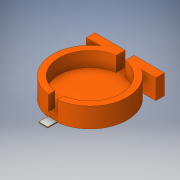
# Autodesk Inventor part: Keystone1056_12_5mmCoinCell
Saved by Autodesk Inventor 2016 (Build 200138000, 138)
## iProperties
Created: 2016-09-29
Part Number: Keystone1056_12_5mmCoinCell
Material: Generic
Document SubType Name: Modeling
Designer: jfixelle
Density: 1 g/cm^3
Appearance: Smooth - Light Orange
Author: jfixelle
Autodesk Inventor part; units mm, degrees
ref_plane "YZ Plane" through (0, 0, 0) normal (1, 0, 0) x (0, 1, 0)
ref_plane "XZ Plane" through (0, 0, 0) normal (0, 1, 0) x (-1, 0, 0)
ref_plane "XY Plane" through (0, 0, 0) normal (0, 0, 1) x (1, 0, 0)
sketch "Sketch1" plane through (0, 0, 0) normal (0, 1, 0) x (-1, 0, 0)
  arc A0 (4.1548, -6.25) -> (-4.1548, -6.25) centre (0, 0) ccw
  circle A1 centre (0, 0) radius 6.25 construction
  line L0 (-7, -6.25) -> (-7, -7.985)
  line L1 (-7, -7.985) -> (7, -7.985)
  line L2 (7, -7.985) -> (7, -6.25)
  line L3 (0, 7.505) -> (-2.894, 7.505)
  line L4 (7, -6.25) -> (4.1548, -6.25)
  line L5 (-4.1548, -6.25) -> (-7, -6.25)
  dimension "d0" = 15.01
  dimension "d1" = 12.5
  dimension "d2" = 15.49
  dimension "d4" = 14
  dimension "d5" = 7
  constraints: 12 end point, 3 horizontal, 3 parallel, 3 point on circle, 2 centre point, 2 coincident, 2 perpendicular, 1 tangent
  measures "d0" diameter of A0
  measures "d1" diameter of A1
  measures "d2" distance between parallel lines of L1 L3
  measures "d4" distance of L0.end L1.end
  measures "d5" distance from line of point (0, 0) L2
extrude "Extrusion1" add sketch "Sketch1" along normal blind 4
sketch "Sketch2" plane through (0, 4, 0) normal (0, 1, 0) x (1, 0, 0)
  circle A0 centre (0, 0) radius 6.25
  line L0 (-0.9, -7.9572) -> (0.9, -7.9572)
  line L1 (0.9, -7.9572) -> (0.9, 8.949)
  line L2 (0.9, 8.949) -> (-0.9, 8.949)
  line L3 (-0.9, 8.949) -> (-0.9, -7.9572)
  dimension "d8" = 12.5
  dimension "d11" = 1.8
  dimension "d12" = 0.9
  constraints: 8 end point, 2 parallel, 1 centre point, 1 coincident, 1 horizontal, 1 perpendicular
  measures "d8" diameter of A0
  measures "d11" distance of L0.start L0.end
  measures "d12" distance from line of point (0, 0) L3
extrude "Extrusion2" cut sketch "Sketch2" against normal blind 3
sketch "Sketch3" plane through (0, 0, 0) normal (0, -1, 0) x (1, 0, 0)
  line L0 (0.9, 5.5692) -> (-0.9, 5.5692)
  line L1 (-0.9, 5.5692) -> (-0.9, 9.4)
  line L2 (-0.9, 9.4) -> (0.9, 9.4)
  line L3 (0.9, 9.4) -> (0.9, 5.5692)
  line L4 (-0.9, -6.2525) -> (0.9, -6.2525)
  line L5 (0.9, -6.2525) -> (0.9, -9.4)
  line L6 (0.9, -9.4) -> (-0.9, -9.4)
  line L7 (-0.9, -9.4) -> (-0.9, -6.2525)
  point P0 (0, 0)
  dimension "d13" = 1.8
  dimension "d14" = 1.8
  dimension "d15" = 0.9
  dimension "d16" = 0.9
  dimension "d17" = 18.8
  dimension "d18" = 9.4
  constraints: 16 end point, 4 parallel, 2 horizontal, 2 perpendicular
  measures "d13" distance of L5.end L6.end
  measures "d14" distance of L1.end L2.end
  measures "d15" distance from line of point (0, 0) L3
  measures "d16" distance from line of point (0, 0) L5
  measures "d17" distance between parallel lines of L6 L2
  measures "d18" distance from line of point (0, 0) L2
extrude "Extrusion3" add sketch "Sketch3" against normal blind 0.2
sketch "Sketch4" plane through (0, 0, 0) normal (0, -1, 0) x (1, 0, 0)
  circle A0 centre (0, -3.51) radius 0.61
  circle A1 centre (0, 3.51) radius 0.455
  point P0 (0, 0)
  dimension "d21" = 3.51
  dimension "d22" = 3.51
  dimension "d23" = 1.22
  dimension "d24" = 0.91
  constraints: 2 centre point
  measures "d21" distance of point (0, 0) A1.centre
  measures "d22" distance of A0.centre point (0, 0)
  measures "d23" diameter of A0
  measures "d24" diameter of A1
extrude "Extrusion4" add sketch "Sketch4" along normal blind 1
body "Solid1"
